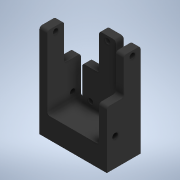
# Autodesk Inventor part: sg_sensor_mount
Saved by Autodesk Inventor 2022 (Build 260153000, 153)
## iProperties
Created: 2022-10-06
Part Number: sg_sensor_mount
Material: Generic
Document SubType Name: Modeling
Designer: janni
Density: 1 g/cm^3
Appearance: Rubber - Black
Author: janni
Autodesk Inventor part; units mm, degrees
ref_plane "YZ Plane" through (0, 0, 0) normal (1, 0, 0) x (0, 1, 0)
ref_plane "TOP" through (0, 36, 0) normal (0, 1, 0) x (-1, 0, 0)
sketch "Sketch1" plane through (0, 0, 0) normal (0, 1, 0) x (-1, 0, 0)
  line L0 (13, -6.5) -> (-13, -6.5)
  line L1 (-13, -6.5) -> (-13, 6.5)
  line L2 (-13, 6.5) -> (13, 6.5)
  line L3 (13, 6.5) -> (13, -6.5)
  line L4 (0, -9.1) -> (0, 9.1) projected
  line L5 (18.2, 0) -> (-18.2, 0) projected
  point P0 (0, 0)
  dimension "d0" = 26
  dimension "d1" = 13
  constraints: 8 end point, 2 parallel, 1 horizontal, 1 perpendicular, 2 other
  measures "d0" distance between parallel lines of L1 L3
  measures "d1" distance between parallel lines of L2 L0
extrude "Extrusion1" add sketch "Sketch1" along normal blind 8
sketch "Sketch2" plane through (0, 8, 0) normal (0, 1, 0) x (1, 0, 0)
  line L0 (-13, 6.5) -> (-13, -6.5) projected
  line L1 (-13, 6.5) -> (-10, 6.5)
  line L2 (-10, 6.5) -> (-10, -6.5)
  line L3 (-10, -6.5) -> (-13, -6.5)
  line L4 (-13, -6.5) -> (-13, 6.5)
  line L5 (13, 6.5) -> (-13, 6.5) projected
  line L6 (13, 6.5) -> (10, 6.5)
  line L7 (10, 6.5) -> (10, -6.5)
  line L8 (10, -6.5) -> (13, -6.5)
  line L9 (13, -6.5) -> (13, 6.5)
  line L10 (-6.5, 6.5) -> (6.5, 6.5)
  line L11 (6.5, 6.5) -> (6.5, 3.5)
  line L12 (6.5, 3.5) -> (-6.5, 3.5)
  line L13 (-6.5, 3.5) -> (-6.5, 6.5)
  line L14 (0, 9.1) -> (0, -9.1) projected
  line L15 (-13, -6.5) -> (13, -6.5) projected
  point P0 (0, 0)
  dimension "d4" = 3
  dimension "d5" = 3
  dimension "d6" = 3
  dimension "d7" = 13
  constraints: 24 end point, 6 parallel, 3 horizontal, 3 perpendicular, 2 point on line, 1 collinear, 1 other
  measures "d4" distance between parallel lines of L12 L5
  measures "d5" distance between parallel lines of L9 L7
  measures "d6" distance between parallel lines of L0 L2
  measures "d7" distance between parallel lines of L11 L13
extrude "Extrusion2" add sketch "Sketch2" along normal up to surface (28 mm away) contours L1 L2 L3 L0 | L5 L14 L12 L13 | L5 L11 L12 L14 | L7 L5 L9 L8
sketch "Sketch3" plane through (-13, 0, -6.5) normal (-1, 0, 0) x (0, 0, 1)
  line L0 (0, 36) -> (6.5, 36)
  line L1 (6.5, 36) -> (6.5, 22)
  line L2 (6.5, 22) -> (0, 22)
  line L3 (0, 22) -> (0, 36)
  line L4 (0, 0) -> (13, 0) projected
  line L5 (13, 0) -> (13, 36) projected
  line L6 (13, 36) -> (0, 36) projected
  line L7 (0, 0) -> (0, 36) projected
  point P0 (6.5, 0)
  dimension "d11" = 22
  dimension "d12" = 6.5
  constraints: 8 end point, 2 collinear, 2 parallel, 1 horizontal, 1 perpendicular
  measures "d11" distance between parallel lines of L2 L4
  measures "d12" distance between parallel lines of L5 L1
extrude "Extrusion3" cut sketch "Sketch3" against normal blind 3 contours L0 L1 L2 L3
sketch "Sketch4" plane through (13, 0, 6.5) normal (1, 0, 0) x (0, 0, -1)
  line L0 (6.5, 36) -> (0, 36) projected
  line L1 (0, 36) -> (6.5, 36)
  line L2 (6.5, 36) -> (6.5, 22)
  line L3 (6.5, 22) -> (0, 22)
  line L4 (0, 22) -> (0, 36)
  line L5 (-2.6, 0) -> (15.6, 0) projected
  line L6 (13, 0) -> (13, 36) projected
  point P0 (6.5, 0)
  dimension "d15" = 22
  dimension "d16" = 6.5
  constraints: 8 end point, 2 parallel, 1 horizontal, 1 perpendicular
  measures "d15" distance between parallel lines of L5 L3
  measures "d16" distance between parallel lines of L2 L6
extrude "Extrusion4" cut sketch "Sketch4" against normal blind 3
sketch "Sketch5" plane through (-6.5, 8, -3.5) normal (0, 0, 1) x (1, 0, 0)
  line L0 (0, 0) -> (0, 28) projected
  line L1 (0, 28) -> (6.5, 28)
  line L2 (6.5, 28) -> (6.5, 14)
  line L3 (6.5, 14) -> (0, 14)
  line L4 (0, 14) -> (0, 28)
  line L5 (13, 0) -> (13, 28) projected
  line L6 (-6.5, -8) -> (19.5, -8) projected
  point P0 (6.5, -8)
  point P1 (0, 14)
  dimension "d19" = 6.5
  dimension "d20" = 22
  constraints: 8 end point, 2 parallel, 1 horizontal, 1 perpendicular
  measures "d19" distance between parallel lines of L2 L5
  measures "d20" distance between parallel lines of L3 L6
extrude "Extrusion5" cut sketch "Sketch5" against normal blind 3
sketch "Sketch6" plane through (13, 0, 6.5) normal (1, 0, 0) x (0, 0, -1)
  circle A0 centre (9.8, 34.2) radius 1.05
  circle A1 centre (3.2, 10.8) radius 1.05
  line L0 (13, 0) -> (13, 36) projected
  line L1 (13, 36) -> (6.5, 36) projected
  line L2 (0, 0) -> (0, 22) projected
  line L3 (6.5, 36) -> (6.5, 22) projected
  point P0 (6.5, 0)
  point P1 (0, 8)
  dimension "d23" = 2.1
  dimension "d25" = 1.8
  dimension "d27" = 2.8
  dimension "d30" = 3.3
  dimension "d31" = 3.3
  constraints: 2 centre point, 1 equal radius
  measures "d23" diameter of A0
  measures "d25" distance from line of A0.centre L1
  measures "d27" vertical distance of A1.centre point (0, 8)
  measures "d30" distance from line of A0.centre L3
  measures "d31" distance from line of A1.centre L3
extrude "Extrusion6" cut sketch "Sketch6" against normal blind 3
ref_plane "Work Plane2" through (13, 22, 6.5) normal (0, 1, 0) x (1, 0, 0)
sketch "Sketch7" plane through (-13, 0, -6.5) normal (-1, 0, 0) x (0, 0, 1)
  circle A0 centre (9.8, 34.2) radius 1
  circle A1 centre (3.2, 10.8) radius 1
  line L0 (6.5, 43.2) -> (6.5, -7.2) projected
  line L1 (13, 36) -> (6.5, 36) projected
  line L2 (13, 8) -> (0, 8) projected
  line L3 (0, 8) -> (3, 8) projected
  line L4 (3, 8) -> (0, 8) projected
  line L5 (0, 8) -> (13, 8) projected
  point P0 (6.5, 0)
  dimension "d33" = 2
  dimension "d34" = 3.3
  dimension "d35" = 1.8
  dimension "d36" = 3.3
  dimension "d37" = 2.8
  constraints: 2 centre point, 1 equal radius
  measures "d33" diameter of A0
  measures "d34" distance from line of A0.centre L0
  measures "d35" distance from line of L1 A0.centre
  measures "d36" distance from line of L0 A1.centre
  measures "d37" distance from line of A1.centre L2
extrude "Extrusion7" cut sketch "Sketch7" against normal blind 3
sketch "Sketch8" plane through (-6.5, 8, -3.5) normal (0, 0, 1) x (1, 0, 0)
  circle A0 centre (9.8, 26.2) radius 1
  circle A1 centre (3.2, 2.8) radius 1
  line L0 (-11.7, 28) -> (24.7, 28) projected
  line L1 (6.5, 35.2) -> (6.5, -15.2) projected
  line L2 (-3.5, 0) -> (16.5, 0) projected
  point P0 (6.5, -8)
  dimension "d40" = 2
  dimension "d41" = 1.8
  dimension "d42" = 3.3
  dimension "d43" = 3.3
  dimension "d44" = 2.8
  constraints: 2 centre point, 1 equal radius
  measures "d40" diameter of A0
  measures "d41" distance from line of A0.centre L0
  measures "d42" distance from line of A0.centre L1
  measures "d43" distance from line of L1 A1.centre
  measures "d44" distance from line of A1.centre L2
extrude "Extrusion8" cut sketch "Sketch8" against normal blind 3
sketch "Sketch9" plane through (0, 0, 0) normal (0, -1, 0) x (1, 0, 0)
  circle A0 centre (-8, 0) radius 2
  circle A1 centre (8, 0) radius 2
  line L0 (0, -9.1) -> (0, 9.1) projected
  line L1 (-18.2, 0) -> (18.2, 0) projected
  point P0 (0, 0)
  dimension "d47" = 4
  dimension "d48" = 16
  constraints: 2 centre point, 1 equal radius, 1 point on line, 1 symmetric about line
  measures "d47" diameter of A0
  measures "d48" distance of A1.centre A0.centre
extrude "Extrusion9" cut sketch "Sketch9" against normal blind 6
fillet "Fillet1" radius 1 11 edges at (10, 8, 0) (-10, 8, 0) (11.5, 22, 6.5) (11.5, 22, 0) (-11.5, 22, -6.5) (-11.5, 22, 0) (-6.5, 22, -5) (0, 22, -5) (6.5, 8, -5) (0, 8, -3.5) (-6.5, 8, -5)
body "Solid1"
